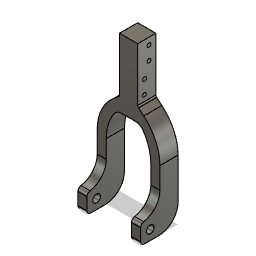
Pedal v1 (Autodesk Fusion 360 design; units mm, degrees)
Autodesk Fusion 360 part; units mm, degrees
sketch "Pedal Shape" plane through (0, 0, 0) normal (0, 0, 1) x (1, 0, 0)
  line L0 (0, 0) -> (0, 89.4421)
  line L1 (0, 89.4421) -> (24.5, 110)
  line L2 (24.5, 110) -> (24.5, 170)
  line L3 (24.5, 170) -> (44.5, 170)
  line L4 (44.5, 170) -> (44.5, 110)
  line L5 (44.5, 110) -> (69, 89.4421)
  line L6 (69, 89.4421) -> (69, 0)
  line L7 (69, 0) -> (59, 0)
  line L8 (59, 0) -> (59, 84.779)
  line L9 (59, 84.779) -> (47.0825, 94.779)
  line L10 (47.0825, 94.779) -> (21.9175, 94.779)
  line L11 (21.9175, 94.779) -> (10, 84.779)
  line L12 (10, 84.779) -> (10, 0)
  line L13 (10, 0) -> (0, 0)
  dimension "d2" = 20
  dimension "d4" = 10
  dimension "d6" = 170
  dimension "d7" = 10
  dimension "d45" = 10
  dimension "d47" = 110
  dimension "d48" = 69
  constraint parallel L0 L2
  constraint perpendicular L2 L3
  constraint perpendicular L3 L4
  constraint perpendicular L3 L6
  constraint perpendicular L6 L7
  constraint perpendicular L7 L8
  constraint parallel L5 L9
  constraint perpendicular L8 L10
  constraint perpendicular L10 L12
  constraint coincident L0.start L13.end
  constraint equal L7 L13
  constraint equal L9 L11
  constraint equal L8 L12
  constraint equal L1 L5
  constraint equal L2 L4
  constraint horizontal L13
  constraint horizontal L7
  constraint collinear L7 L13
  constraint parallel L1 L11
  measures "d2" distance of L2.end L3.end
  measures "d4" distance of L0 L12
  measures "d6" distance of L3 L13
  measures "d7" distance of L5 L9
  measures "d45" distance of L10 L11.end
  measures "d47" distance of L1.end L13
  measures "d48" distance of L0 L6
extrude "Extrude1" add sketch "Pedal Shape" along normal blind 20
sketch "Pivot Point" plane through (0, 0, 0) normal (-1, 0, 0) x (0, 0, 1)
  line L0 (0, 89.4421) -> (0, 0)
  line L1 (0, 0) -> (20, 0)
  line L2 (20, 0) -> (20, 89.4421)
  line L3 (20, 89.4421) -> (0, 89.4421)
  circle A0 centre (30.625, 10.625) radius 4.25
  line L4 (20, 21.25) -> (41.25, 21.25)
  line L5 (41.25, 21.25) -> (41.25, 0)
  line L6 (41.25, 0) -> (20, 0)
  line L7 (20, 21.25) -> (20, 0)
  line L8 (30.625, 21.25) -> (30.625, 0) construction
  dimension "d12" = 8.5
  dimension "d13" = 10.625
  dimension "d16" = 21.25
  dimension "d17" = 21.25
  constraint coincident L2 L4.start
  constraint perpendicular L2 L4
  constraint perpendicular L4 L5
  constraint coincident L1.end L2.start
  constraint perpendicular L2 L6
  constraint midpoint L4 L8.start
  constraint midpoint L6 L8.end
  constraint coincident A0.centre L8
  measures "d12" diameter of A0
  measures "d13" distance of L1 A0.centre
  measures "d16" distance of L4.end L5.end
  measures "d17" distance of L5 L7
extrude "Extrude3" add sketch "Pivot Point" against normal blind 10 contours L2 L4 L5 L6 L7
fillet "Fillet1" radius 21.25 1 edges at (5, 21.25, 20)
fillet "Fillet1" radius 21.25 1 edges at (5, 0, 0)
ref_plane "WorkPlane1" through (34.5, 44.721, 10) normal (1, 0, 0) x (0, 1, 0)
mirror "Mirror1" about plane through (34.5, 44.721, 10) normal (1, 0, 0) of "Extrude3", "Fillet1"
sketch "Pedal and Connector Holes" plane through (44.5, 0, 0) normal (1, 0, 0) x (0, 0, -1)
  line L0 (0, 110) -> (0, 170)
  line L1 (0, 170) -> (-20, 170)
  line L2 (-20, 170) -> (-20, 110)
  line L3 (-20, 110) -> (0, 110)
  circle A0 centre (-12.5, 117.5) radius 2.125
  circle A1 centre (-12.5, 132.5) radius 2.125
  line L4 (-12.5, 105) -> (-12.5, 132.5) construction
  circle A2 centre (-7.5, 162.5) radius 2.125
  circle A3 centre (-7.5, 147.5) radius 2.125
  line L5 (-7.5, 162.5) -> (-7.5, 147.5) construction
  dimension "d27" = 4.25
  dimension "d28" = 4.25
  dimension "d29" = 15
  dimension "d30" = 7.5
  dimension "d33" = 7.5
  dimension "d34" = 4.25
  dimension "d35" = 4.25
  dimension "d36" = 15
  dimension "d37" = 7.5
  dimension "d38" = 7.5
  constraint coincident A1.centre L4.end
  constraint coincident A0.centre L4
  constraint vertical L4
  constraint coincident A2.centre L5.start
  constraint coincident A3.centre L5.end
  constraint vertical L5
  measures "d27" diameter of A0
  measures "d28" diameter of A1
  measures "d29" distance of A0.centre A1.centre
  measures "d30" distance of L3 A0.centre
  measures "d33" distance of L2 L4
  measures "d34" diameter of A3
  measures "d35" diameter of A2
  measures "d36" distance of A2.centre A3.centre
  measures "d37" distance of L0 A2.centre
  measures "d38" distance of L1 A2.centre
extrude "Extrude4" cut sketch "Pedal and Connector Holes" against normal up to surface (20 mm away) contours A0 | A1 | A2 | A3
fillet "Fillet2" radius 50 4 edges at (59, 84.779, 10) (10, 84.779, 10) (0, 89.4421, 10) (69, 89.4421, 10)
fillet "Fillet3" radius 10 2 edges at (47.0825, 94.779, 10) (21.9175, 94.779, 10)
fillet "Fillet4" radius 2.5 2 edges at (24.5, 110, 10) (44.5, 110, 10)
fillet "Fillet5" radius 4 4 edges at (64, 21.25, 41.25) (64, 0, 41.25) (5, 0, 41.25) (5, 21.25, 41.25)
equation "d13 = d12 * 1.25"
equation "d16 = d12 * 2.5"
equation "d17 = d16"
equation "d21 = d17"
equation "d23 = d17"
equation "d26 = -d4"
equation "d36 = d29"
equation "d37 = d33"
equation "d38 = d30"
